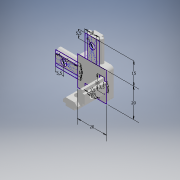
# Autodesk Inventor part: corner
Saved by Autodesk Inventor 2018 (Build 220112000, 112)
## iProperties
Created: 2018-05-23
Part Number: corner
Material: Generic
Document SubType Name: Modeling
Designer: Z. Deniz
Density: 1 g/cm^3
Appearance: Default
Author: Z. Deniz
Autodesk Inventor part; units mm, degrees
ref_plane "YZ Plane" through (0, 0, 0) normal (1, 0, 0) x (0, 1, 0)
ref_plane "XZ Plane" through (0, 0, 0) normal (0, 1, 0) x (-1, 0, 0)
ref_plane "XY Plane" through (0, 0, 0) normal (0, 0, 1) x (1, 0, 0)
sketch "Sketch2" plane through (0, 0, 0) normal (0, 1, 0) x (-1, 0, 0)
  line L0 (0, 0) -> (-20, 0)
  line L1 (-20, 0) -> (-20, -20)
  line L2 (-20, -20) -> (0, -20)
  line L3 (0, -20) -> (0, 0)
  line L4 (-10, 0) -> (-10, 15) construction
  line L5 (-5, 0) -> (-15, 0)
  line L6 (-15, 0) -> (-15, 15)
  line L7 (-15, 15) -> (-5, 15)
  line L8 (-5, 15) -> (-5, 0)
  line L9 (-5, 0) -> (-15, 15) construction
  line L10 (-15, 0) -> (-5, 15) construction
  line L11 (0, -10) -> (15, -10) construction
  line L12 (15, -15) -> (0, -15)
  line L13 (0, -15) -> (0, -5)
  line L14 (0, -5) -> (15, -5)
  line L15 (15, -5) -> (15, -15)
  line L16 (15, -15) -> (0, -5) construction
  line L17 (0, -15) -> (15, -5) construction
  line L18 (15, -13) -> (0, -13)
  line L19 (0, -13) -> (0, -7)
  line L20 (0, -7) -> (15, -7)
  line L21 (15, -7) -> (15, -13)
  line L22 (15, -13) -> (0, -7) construction
  line L23 (0, -13) -> (15, -7) construction
  line L24 (-7, 0) -> (-13, 0)
  line L25 (-13, 0) -> (-13, 15)
  line L26 (-13, 15) -> (-7, 15)
  line L27 (-7, 15) -> (-7, 0)
  line L28 (-7, 0) -> (-13, 15) construction
  line L29 (-13, 0) -> (-7, 15) construction
  line L30 (-10, -20) -> (-10, -18.5) construction
  line L31 (-7, -18.5) -> (-13, -18.5)
  line L32 (-13, -18.5) -> (-13, -20)
  line L33 (-13, -20) -> (-7, -20)
  line L34 (-7, -20) -> (-7, -18.5)
  line L35 (-7, -18.5) -> (-13, -20) construction
  line L36 (-13, -18.5) -> (-7, -20) construction
  line L37 (-10, -18.5) -> (-10, -15) construction
  line L38 (-5, -15) -> (-15, -15)
  line L39 (-15, -15) -> (-15, -18.5)
  line L40 (-15, -18.5) -> (-5, -18.5)
  line L41 (-5, -18.5) -> (-5, -15)
  line L42 (-5, -15) -> (-15, -18.5) construction
  line L43 (-15, -15) -> (-5, -18.5) construction
  line L44 (-20, -10) -> (-18.5, -10) construction
  line L45 (-18.5, -10) -> (-15, -10) construction
  line L46 (-15, -15) -> (-18.5, -15)
  line L47 (-18.5, -15) -> (-18.5, -5)
  line L48 (-18.5, -5) -> (-15, -5)
  line L49 (-15, -5) -> (-15, -15)
  line L50 (-15, -15) -> (-18.5, -5) construction
  line L51 (-18.5, -15) -> (-15, -5) construction
  line L52 (-18.5, -13) -> (-20, -13)
  line L53 (-20, -13) -> (-20, -7)
  line L54 (-20, -7) -> (-18.5, -7)
  line L55 (-18.5, -7) -> (-18.5, -13)
  line L56 (-18.5, -13) -> (-20, -7) construction
  line L57 (-20, -13) -> (-18.5, -7) construction
  circle A0 centre (-10, 9.5) radius 2
  circle A1 centre (9.5, -10) radius 2
  point P0 (-10, 7.5)
  point P1 (7.5, -10)
  point P2 (-10, -19.25)
  point P3 (-10, -16.75)
  point P4 (-16.75, -10)
  point P5 (-19.25, -10)
  dimension "d0" = 20
  dimension "d1" = 20
  dimension "d2" = 15
  dimension "d3" = 10
  dimension "d4" = 15
  dimension "d5" = 10
  dimension "d6" = 6
  dimension "d7" = 6
  dimension "d8" = 1.5
  dimension "d9" = 6
  dimension "d10" = 3.5
  dimension "d11" = 10
  dimension "d18" = 1.5
  dimension "d19" = 3.5
  dimension "d20" = 10
  dimension "d21" = 6
  dimension "d38" = 4
  dimension "d39" = 5.5
  dimension "d40" = 4
  dimension "d41" = 5.5
  constraints: 116 end point, 26 midpoint, 18 parallel, 13 horizontal, 9 perpendicular, 8 point on line, 4 vertical, 2 centre point
  measures "d0" distance of L2.end L1.end
  measures "d1" distance of L1.end L0.end
  measures "d2" distance of L4.start L4.end
  measures "d3" distance of L6.end L7.end
  measures "d4" distance of L11.start L11.end
  measures "d5" distance of L12.end L13.end
  measures "d6" distance of L18.end L19.end
  measures "d7" distance of L25.end L26.end
  measures "d8" distance of L30.start L30.end
  measures "d9" distance of L33.end L32.end
  measures "d10" distance of L30.end L37.end
  measures "d11" distance of L40.end L39.end
  measures "d18" distance of L44.start L44.end
  measures "d19" distance of L44.end L45.end
  measures "d20" distance of L46.end L47.end
  measures "d21" distance of L52.end L53.end
  measures "d38" diameter of A0
  measures "d39" distance from line of L7 A0.centre
  measures "d40" diameter of A1
  measures "d41" distance from line of L15 A1.centre
extrude "Extrusion3" add sketch "Sketch2" along normal blind 3.5 contours L0 L27 L7 L8 | L14 L15 L20 L3 | L0 L6 L7 L25 | L18 L15 L12 L3
extrude "Extrusion4" add sketch "Sketch2" along normal blind 5 contours L3 L2 L34 L40 L41 L38 L49 L48 L47 L54 L1 L0 | L0 L25 L7 L27 | L20 L15 L18 L3 | L54 L47 L52 L1 | L2 L32 L31 L34 | L52 L47 L46 L39 L40 L32 L2 L1 | L47 L48 L49 L46 | L31 L40 L39 L38 L41
extrude "Extrusion5" add sketch "Sketch2" against normal blind 15 contours L2 L32 L31 L34 | L31 L40 L39 L38 L41
fillet "Fillet1" radius 2 4 edges at (0, 2.5, -20) (0, 2.5, 0) (20, 2.5, 0) (20, 2.5, -20)
chamfer "Chamfer1" distance 2 angle 45 5 edges at (-7.5, 0, -5) (-7.5, 0, -15) (5, 0, 7.5) (15, 0, 7.5) (5, -7.5, -15)
chamfer "Chamfer2" distance 2 angle 45 1 edges at (15, -7.5, -15)
extrude "Extrusion6" add sketch "Sketch2" against normal blind 15 contours L54 L47 L52 L1 | L47 L48 L49 L46
chamfer "Chamfer3" distance 2 angle 45 2 edges at (15, -7.5, -5) (15, -7.5, -15)
sketch "Sketch3" plane through (20, 0, -18) normal (1, 0, 0) x (0, 0, -1)
  circle A0 centre (-8, -9.5) radius 2
  line L0 (-5, -15) -> (-11, -15) projected
  line L1 (-5, 0) -> (-5, -15) projected
  point P0 (-18, 0)
  dimension "d42" = 4
  dimension "d43" = 5.5
  dimension "d51" = 3
  constraints: 1 centre point
  measures "d42" diameter of A0
  measures "d43" distance from line of L0 A0.centre
  measures "d51" distance from line of L1 A0.centre
extrude "Extrusion7" cut sketch "Sketch3" against normal blind 5
sketch "Sketch4" plane through (13, -15, -20) normal (0, 0, -1) x (-1, 0, 0)
  circle A0 centre (3, 5.5) radius 2
  line L0 (6, 0) -> (0, 0) projected
  line L1 (6, 15) -> (6, 0) projected
  point P0 (13, 15)
  dimension "d46" = 4
  dimension "d47" = 5.5
  dimension "d48" = 3
  constraints: 1 centre point
  measures "d46" diameter of A0
  measures "d47" distance from line of L0 A0.centre
  measures "d48" distance from line of L1 A0.centre
extrude "Extrusion8" cut sketch "Sketch4" against normal blind 5
body "Solid1"
